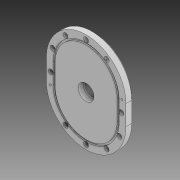
# Autodesk Inventor part: housingPlate
Saved by Autodesk Inventor 2020 (Build 240168000, 168)
## iProperties
Created: 2020-11-25
Part Number: housingPlate
Material: Generic
Document SubType Name: Modeling
Designer: DDeGo
Density: 1 g/cm^3
Appearance: Default
Author: DDeGo
Autodesk Inventor part; units mm, degrees
ref_plane "YZ Plane" through (0, 0, 0) normal (1, 0, 0) x (0, 1, 0)
ref_plane "XZ Plane" through (0, 0, 0) normal (0, 1, 0) x (-1, 0, 0)
ref_plane "XY Plane" through (0, 0, 0) normal (0, 0, 1) x (1, 0, 0)
sketch "Sketch1" plane through (0, 0, 0) normal (0, 0, 1) x (1, 0, 0)
  line L0 (0, 0) -> (0, 5.2) construction
  arc A0 (15.6034, 1.2322) -> (-15.6034, 1.2322) centre (0, 5.2) ccw construction
  line L1 (0, 0) -> (0, -5.2) construction
  arc A1 (-15.6034, -1.2322) -> (15.6034, -1.2322) centre (0, -5.2) ccw construction
  line L2 (0, 5.2) -> (0, -5.2) construction
  line L3 (-20.7, 5.2) -> (-20.7, -5.2)
  line L4 (20.7, -5.2) -> (20.7, 5.2)
  arc A2 (20.7, 5.2) -> (-20.7, 5.2) centre (0, 5.2) ccw
  arc A3 (-20.7, -5.2) -> (20.7, -5.2) centre (0, -5.2) ccw
  arc A4 (-15.6034, -1.2322) -> (-15.6034, 1.2322) centre (-20.4492, 0) ccw construction
  arc A5 (15.6034, 1.2322) -> (15.6034, -1.2322) centre (20.4492, 0) ccw construction
  line L5 (0, 5.2) -> (0, -5.2) construction
  circle A6 centre (0, 0) radius 14.5 construction
  dimension "d0" = 10.4
  dimension "d1" = 16.1
  dimension "d2" = 4.6
  dimension "d3" = 5
  dimension "d4" = 41.4
  dimension "d8" = 29
  constraints: 16 end point, 12 point on circle, 8 tangent, 7 centre point, 4 coincident, 3 vertical, 2 collinear, 2 equal radius, 2 midpoint, 1 parallel
  measures "d0" distance of L1.end L0.end
  measures "d1" radius of A0
  measures "d2" radial gap between concentric circles of A3 A1
  measures "d3" radius of A4
  measures "d4" distance between parallel lines of L4 L3
  measures "d8" diameter of A6
extrude "Extrusion1" add sketch "Sketch1" along normal blind 4
sketch "Sketch2" plane through (0, 0, 4) normal (0, 0, 1) x (1, 0, 0)
  line L0 (-20.7, 5.2) -> (-20.7, -5.2) construction
  arc A0 (-20.7, -5.2) -> (20.7, -5.2) centre (0, -5.2) ccw construction
  line L1 (20.7, -5.2) -> (20.7, 5.2) construction
  arc A1 (20.7, 5.2) -> (-20.7, 5.2) centre (0, 5.2) ccw construction
  line L2 (-18.4, 5.2) -> (-18.4, -5.2) construction
  arc A2 (-18.4, -5.2) -> (18.4, -5.2) centre (0, -5.2) ccw construction
  line L3 (18.4, -5.2) -> (18.4, 5.2) construction
  arc A3 (18.4, 5.2) -> (-18.4, 5.2) centre (0, 5.2) ccw construction
  circle A4 centre (-18.4, 0) radius 1.25
  circle A5 centre (0, 23.6) radius 1.25
  circle A6 centre (-10.6895, 20.1765) radius 1.25
  circle A7 centre (-17.4012, 11.1798) radius 1.25
  line L4 (-18.4, 0) -> (-17.4012, 11.1798) construction
  line L5 (-17.4012, 11.1798) -> (-10.6895, 20.1765) construction
  line L6 (-10.6895, 20.1765) -> (0, 23.6) construction
  line L7 (-18.4, 0) -> (0, 0) construction
  line L8 (0, 0) -> (0, 23.6) construction
  circle A8 centre (18.4, 0) radius 1.25
  circle A9 centre (10.6895, 20.1765) radius 1.25
  circle A10 centre (17.4012, 11.1798) radius 1.25
  circle A11 centre (0, -23.6) radius 1.25
  circle A12 centre (-10.6895, -20.1765) radius 1.25
  circle A13 centre (-17.4012, -11.1798) radius 1.25
  circle A14 centre (10.6895, -20.1765) radius 1.25
  circle A15 centre (17.4012, -11.1798) radius 1.25
  line L9 (-18.4, 0) -> (-18.4, -6) construction
  line L10 (-18.4, -6) -> (-18.628, -6) construction
  line L11 (18.4, 0) -> (18.4, 6) construction
  line L12 (18.4, 6) -> (18.628, 6) construction
  circle A16 centre (-18.628, -6) radius 0.5
  circle A17 centre (18.628, 6) radius 0.5
  dimension "d37" = 2.3
  dimension "d38" = 2.5
  dimension "d39" = 6
  dimension "d40" = 0.228
  dimension "d41" = 6
  dimension "d42" = 0.228
  dimension "d43" = 1
  constraints: 22 end point, 16 centre point, 8 symmetric about line, 7 point on circle, 4 equal radius, 3 perpendicular, 2 coincident, 2 equal length, 2 point on line, 1 horizontal, 1 midpoint, 11 other
  measures "d37" distance between parallel lines of L1 L3
  measures "d38" diameter of A4
  measures "d39" distance of L4.start L9.end
  measures "d40" distance of L9.end L10.end
  measures "d41" distance of L11.start L11.end
  measures "d42" distance of L11.end L12.end
  measures "d43" diameter of A16
extrude "Extrusion2" cut sketch "Sketch2" against normal through all contours A4 | A5 | A6 | A7 | A8 | A9 | A11 | A12 | A14 | A15 | A16 | A17
sketch "Sketch5" plane through (0, 0, 4) normal (0, 0, 1) x (1, 0, 0)
  line L0 (20.7, -5.2) -> (20.7, 5.2) construction
  arc A0 (20.7, 5.2) -> (-20.7, 5.2) centre (0, 5.2) ccw construction
  line L1 (-20.7, 5.2) -> (-20.7, -5.2) construction
  arc A1 (-20.7, -5.2) -> (20.7, -5.2) centre (0, -5.2) ccw construction
  arc A2 (17.15, 5.2) -> (-17.15, 5.2) centre (0, 5.2) ccw
  line L2 (17.15, 5.2) -> (17.15, -5.2)
  arc A3 (-17.15, -5.2) -> (17.15, -5.2) centre (0, -5.2) ccw
  line L3 (-17.15, -5.2) -> (-17.15, 5.2)
  arc A4 (16.15, 5.2) -> (-16.15, 5.2) centre (0, 5.2) ccw
  line L4 (16.15, 5.2) -> (16.15, -5.2)
  arc A5 (-16.15, -5.2) -> (16.15, -5.2) centre (0, -5.2) ccw
  line L5 (-16.15, -5.2) -> (-16.15, 5.2)
  point P0 (0, 0)
  dimension "d20" = 1
  constraints: 8 end point, 8 point on circle, 4 centre point, 6 other
  measures "d20" radial gap between concentric circles of A4 A2
extrude "Extrusion5" cut sketch "Sketch5" against normal blind 0.7
fillet "Fillet1" [suppressed]
chamfer "Chamfer1" distance 1 angle 45 4 edges at (0, -25.9, 0) (20.7, 0, 0) (0, 25.9, 0) (-20.7, 0, 0)
sketch "Sketch8" plane through (0, 0, 0) normal (1, 0, 0) x (0, 1, 0)
  line L0 (0, 0) -> (5.2, 0) construction
  line L1 (0, 0) -> (0, 0.9) construction
  line L2 (-5.2, 4) -> (5.2, 4) construction
  line L3 (0, 4) -> (4.075, 4)
  line L4 (4.075, 4) -> (4.075, 1.4)
  line L5 (4.075, 1.4) -> (3.575, 0.9)
  line L6 (3.575, 0.9) -> (0, 0.9)
  line L7 (0, 0.9) -> (0, 4)
  dimension "d44" = 4.075
  dimension "d45" = 135
  dimension "d46" = 2.6
  dimension "d47" = 0.5
  dimension "d48" = 0.9
  constraints: 12 end point, 3 perpendicular, 1 horizontal, 1 midpoint
  measures "d44" distance between parallel lines of L7 L4
  measures "d45" angle of L4 L5
  measures "d46" distance of L3.end L4.end
  measures "d47" distance from line of L4.end L6
  measures "d48" distance between parallel lines of L6 L0
revolve "Revolution1" cut sketch "Sketch8" angle 360 about axis through (0, 0, 0.9) along (0, 0, 1)
sketch "Sketch9" plane through (0, 0, 0) normal (0, 0, -1) x (-1, 0, 0)
  circle A0 centre (-18.628, 6) radius 0.5 projected
  circle A1 centre (18.628, -6) radius 0.5 projected
  point P0 (0, 0)
extrude "Extrusion8" add sketch "Sketch9" against normal blind 0.8
body "Solid1"
